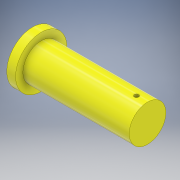
# Autodesk Inventor part: Perno
Saved by Autodesk Inventor 2018 (Build 220112000, 112)
## iProperties
Created: 2020-01-29
Part Number: Perno
Material: Plástico PC/ABS
Document SubType Name: Modeling
Designer: aidan
Density: 0.357273 g/cm^3
Appearance: Suave - Blanco
Author: aidan
Autodesk Inventor part; units mm, degrees
ref_plane "YZ Plane" through (0, 0, 0) normal (1, 0, 0) x (0, 1, 0)
ref_plane "XZ Plane" through (0, 0, 0) normal (0, 1, 0) x (-1, 0, 0)
ref_plane "XY Plane" through (0, 0, 0) normal (0, 0, 1) x (1, 0, 0)
sketch "Boceto1" plane through (0, 0, 0) normal (0, 0, 1) x (1, 0, 0)
  line L0 (0, 0) -> (157, 0)
  line L1 (157, 0) -> (157, 25)
  line L2 (157, 25) -> (12, 25)
  line L3 (0, 0) -> (0, 35)
  line L4 (0, 35) -> (12, 35)
  line L5 (12, 35) -> (12, 25)
  dimension "d1" = 25
  dimension "d2" = 35
  dimension "d3" = 12
  dimension "d4" = 157
  constraints: 12 end point, 2 horizontal, 2 perpendicular, 1 parallel, 1 vertical
  measures "d1" distance of L1.end L0.end
  measures "d2" distance of L0.start L3.end
  measures "d3" distance of L3.end L4.end
  measures "d4" distance between parallel lines of L3 L1
revolve "Revolución1" add sketch "Boceto1" angle 360 about axis through (0, 0, 0) along (1, 0, 0)
sketch "Boceto2" plane through (0, 0, 0) normal (0, 0, 1) x (1, 0, 0)
  circle A0 centre (142, 0) radius 3
  line L0 (12, -35) -> (12, 35) projected
  point P0 (0, 0)
  dimension "d6" = 6
  dimension "d7" = 130
  constraints: 1 centre point
  measures "d6" diameter of A0
  measures "d7" distance from line of L0 A0.centre
extrude "Extrusión1" cut sketch "Boceto2" against normal blind 30 and the other way blind 30
